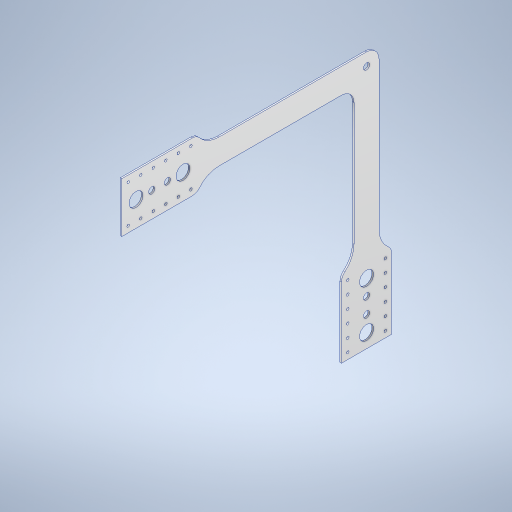
# Autodesk Inventor part: L3Plate
Saved by Autodesk Inventor 2023 (Build 270158000, 158)
## iProperties
Created: 2023-02-05
Part Number: L3Plate
Material: Aluminum 6061
Document SubType Name: Modeling
Designer: Dave
Density: 2.7 g/cm^3
Appearance: Aluminum - Flat
Mass: 543.403 g
Surface Area: 1367.92 cm^2
Volume: 201.26 cm^3
Author: Dave
Autodesk Inventor part; units mm, degrees
ref_plane "YZ Plane" through (0, 0, 0) normal (1, 0, 0) x (0, 1, 0)
ref_plane "XZ Plane" through (0, 0, 0) normal (0, 1, 0) x (-1, 0, 0)
ref_plane "XY Plane" through (0, 0, 0) normal (0, 0, 1) x (1, 0, 0)
sketch "Sketch1" plane through (0, 0, 0) normal (1, 0, 0) x (0, 1, 0)
  line L0 (0, 0) -> (101.6, 0)
  line L1 (101.6, 0) -> (101.6, -152.4)
  line L2 (101.6, -152.4) -> (0, -152.4)
  line L3 (0, -152.4) -> (0, 0)
  circle A0 centre (50.8, -28.575) radius 14.2875
  circle A1 centre (50.8, -60.325) radius 6.35
  circle A2 centre (50.8, -92.075) radius 6.35
  circle A3 centre (50.8, -123.825) radius 14.2875
  line L4 (50.8, -28.575) -> (50.8, -123.825) construction
  circle A4 centre (88.9, -12.7) radius 2.65
  circle A5 centre (88.9, -38.1) radius 2.65
  circle A6 centre (88.9, -63.5) radius 2.65
  circle A7 centre (88.9, -88.9) radius 2.65
  circle A8 centre (88.9, -114.3) radius 2.65
  circle A9 centre (88.9, -139.7) radius 2.65
  circle A10 centre (12.7, -12.7) radius 2.65
  circle A11 centre (12.7, -38.1) radius 2.65
  circle A12 centre (12.7, -63.5) radius 2.65
  circle A13 centre (12.7, -88.9) radius 2.65
  circle A14 centre (12.7, -114.3) radius 2.65
  circle A15 centre (12.7, -139.7) radius 2.65
  line L5 (76.2, -152.4) -> (76.2, -508.635)
  line L6 (25.4, -470.535) -> (25.4, -152.4)
  circle A16 centre (50.8, -495.935) radius 6.35
  line L7 (50.8, -495.935) -> (-491.6426, 46.5076) construction
  line L8 (50.8, -495.935) -> (817.9296, -495.935) construction
  line L9 (-445.135, -546.735) -> (-292.735, -546.735)
  line L10 (-292.735, -546.735) -> (-292.735, -445.135)
  line L11 (-292.735, -445.135) -> (-445.135, -445.135)
  circle A17 centre (-416.56, -495.935) radius 14.2875
  circle A18 centre (-384.81, -495.935) radius 6.35
  circle A19 centre (-353.06, -495.935) radius 6.35
  circle A20 centre (-321.31, -495.935) radius 14.2875
  line L12 (-416.56, -495.935) -> (-321.31, -495.935) construction
  circle A21 centre (-432.435, -534.035) radius 2.65
  circle A22 centre (-407.035, -534.035) radius 2.65
  circle A23 centre (-381.635, -534.035) radius 2.65
  circle A24 centre (-356.235, -534.035) radius 2.65
  circle A25 centre (-330.835, -534.035) radius 2.65
  circle A26 centre (-305.435, -534.035) radius 2.65
  circle A27 centre (-432.435, -457.835) radius 2.65
  circle A28 centre (-407.035, -457.835) radius 2.65
  circle A29 centre (-381.635, -457.835) radius 2.65
  circle A30 centre (-356.235, -457.835) radius 2.65
  circle A31 centre (-330.835, -457.835) radius 2.65
  circle A32 centre (-305.435, -457.835) radius 2.65
  line L13 (-292.735, -521.335) -> (63.5, -521.335)
  line L14 (25.4, -470.535) -> (-292.735, -470.535)
  circle A33 centre (50.8, -495.935) radius 6.35
  line L15 (50.8, -495.935) -> (50.8, -1263.0646) construction
  line L16 (76.2, -521.335) -> (63.5, -521.335)
  line L17 (76.2, -508.635) -> (76.2, -521.335)
  line L18 (-445.135, -445.135) -> (-445.135, -546.735)
  point P0 (101.6, -76.2)
  point P1 (50.8, -76.2)
  point P2 (50.8, -152.4)
  point P3 (-368.935, -546.735)
  point P4 (-368.935, -495.935)
  point P5 (-292.735, -495.935)
  point P6 (63.5, -470.535)
  dimension "d0" = 101.6
  dimension "d1" = 152.4
  dimension "d2" = 28.575
  dimension "d3" = 12.7
  dimension "d4" = 12.7
  dimension "d5" = 28.575
  dimension "d6" = 31.75
  dimension "d7" = 31.75
  dimension "d8" = 31.75
  dimension "d9" = 5.3
  dimension "d10" = 12.7
  dimension "d11" = 12.7
  dimension "d14" = 25.4
  dimension "d17" = 76.2
  dimension "d22" = 12.7
  dimension "d24" = 467.36
  dimension "d25" = 25.4
  dimension "d26" = 50.8
  dimension "d27" = 135
  constraints: 38 end point, 34 centre point, 27 symmetric about line, 7 point on line, 4 horizontal, 4 vertical alignment, 3 midpoint, 3 perpendicular, 3 vertical, 2 parallel, 1 equal length, 1 horizontal alignment, 39 other
  measures "d0" distance of L1.end L2.end
  measures "d1" distance of L0.end L1.end
  measures "d2" diameter of A0
  measures "d3" diameter of A1
  measures "d4" diameter of A2
  measures "d5" diameter of A3
  measures "d6" distance of A1.centre L4.start
  measures "d7" distance of A2.centre A1.centre
  measures "d8" distance of A2.centre L4.end
  measures "d9" diameter of A4
  measures "d10" distance from line of L1 A4.centre
  measures "d11" distance from line of L0 A4.centre
  measures "d14" distance of A4.centre A5.centre
  measures "d17" distance of A4.centre A10.centre
  measures "d22" diameter of A16
  measures "d24" distance of L7.start L4.start
  measures "d25" distance between parallel lines of L4 L5
  measures "d26" distance between parallel lines of L5 L6
  measures "d27" angle of L8 L7
extrude "Extrusion1" add sketch "Sketch1" along normal blind 3.175
fillet "Fillet1" radius 50.8 4 edges at (1.5875, 76.2, -152.4) (1.5875, 25.4, -152.4) (1.5875, -292.735, -470.535) (1.5875, -292.735, -521.335)
fillet "Fillet2" radius 25.4 2 edges at (1.5875, 76.2, -521.335) (1.5875, 25.4, -470.535)
fillet "Fillet3" radius 19.05 4 edges at (1.5875, 101.6, -152.4) (1.5875, 0, -152.4) (1.5875, -292.735, -445.135) (1.5875, -292.735, -546.735)
equation "\"d7\" = d6"
equation "\"d8\" = d7"
body "Solid1"
